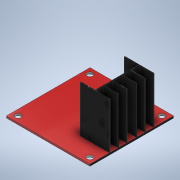
# Autodesk Inventor part: L298N
Saved by Autodesk Inventor 2022 (Build 260153000, 153)
## iProperties
Created: 2022-02-10
Part Number: L298N
Material: Generic
Document SubType Name: Modeling
Designer: matys
Density: 1 g/cm^3
Appearance: Default
Author: matys
Autodesk Inventor part; units mm, degrees
ref_plane "YZ Plane" through (0, 0, 0) normal (1, 0, 0) x (0, 1, 0)
ref_plane "XZ Plane" through (0, 0, 0) normal (0, 1, 0) x (-1, 0, 0)
ref_plane "XY Plane" through (0, 0, 0) normal (0, 0, 1) x (1, 0, 0)
sketch "Sketch1" plane through (0, 0, 0) normal (0, 1, 0) x (-1, 0, 0)
  line L0 (0, 0) -> (0, -43)
  line L1 (0, -43) -> (43, -43)
  line L2 (43, -43) -> (43, 0)
  line L3 (43, 0) -> (0, 0)
  dimension "d0" = 43
  dimension "d1" = 43
  constraints: 8 end point, 3 perpendicular, 1 vertical
  measures "d0" distance of L0.start L0.end
  measures "d1" distance of L0.end L1.end
extrude "Extrusion1" add sketch "Sketch1" along normal blind 1
sketch "Sketch2" plane through (0, 1, 0) normal (0, 1, 0) x (1, 0, 0)
  line L0 (-43, 0) -> (0, 0) projected
  line L1 (0, 0) -> (-3, 0)
  line L2 (-3, 0) -> (-3, 3)
  line L3 (-3, 3) -> (0, 3)
  circle A0 centre (-3, 3) radius 1.5
  line L4 (0, 43) -> (-43, 43) projected
  line L5 (0, 0) -> (-43, 43)
  line L6 (-43, 43) -> (-43, 0)
  line L7 (-43, 43) -> (-43, 0) projected
  line L8 (0, 0) -> (0, 43) projected
  line L9 (-43, 0) -> (0, 43)
  line L10 (0, 43) -> (-21.5, 21.5)
  circle A1 centre (-3, 40) radius 1.5
  circle A2 centre (-40, 40) radius 1.5
  circle A3 centre (-40, 3) radius 1.5
  dimension "d4" = 3
  dimension "d5" = 3
  dimension "d6" = 3
  dimension "d9" = 360
  constraints: 14 end point, 4 centre point, 4 perpendicular, 1 coincident, 1 midpoint, 1 point on line, 9 other
  measures "d4" distance of L0.end L1.end
  measures "d5" distance of L1.end L2.end
  measures "d6" diameter of A0
extrude "Extrusion2" cut sketch "Sketch2" against normal through all contours A3 L9 | L9 A3 | A0 L5 L2 | L2 L5 A0 | A2 L5 | L5 A2 | L5 L3 A0 | L5 A0 L3 | A1 L9 | L9 A1
sketch "Sketch3" plane through (0, 1, 0) normal (0, 1, 0) x (1, 0, 0)
  line L0 (-43, 0) -> (0, 0) projected
  line L1 (0, 0) -> (0, 10)
  line L2 (0, 0) -> (0, 43) projected
  line L3 (0, 10) -> (0, 43)
  line L4 (0, 43) -> (0, 33)
  line L5 (0, 33) -> (0, 10)
  line L6 (0, 10) -> (-15, 10)
  line L7 (-15, 10) -> (-15, 33)
  line L8 (-15, 33) -> (0, 33)
  line L9 (0, 10) -> (0, 14.4)
  line L10 (0, 14.4) -> (0, 18.8)
  line L11 (0, 33) -> (0, 28.6)
  line L12 (0, 28.6) -> (0, 24.2)
  line L13 (0, 24.2) -> (0, 18.8)
  line L14 (0, 14.4) -> (0, 15)
  line L15 (0, 33) -> (0, 32.6)
  line L16 (0, 32.6) -> (-15, 32.6)
  line L17 (0, 32.6) -> (0, 28.6)
  line L18 (0, 28.6) -> (-15, 28.6)
  line L19 (0, 28.6) -> (0, 28.2)
  line L20 (0, 28.2) -> (-15, 28.2)
  line L21 (0, 28.2) -> (0, 24.2)
  line L22 (0, 18.8) -> (0, 24.2)
  line L23 (0, 32.6) -> (0, 28.6)
  line L24 (0, 28.2) -> (0, 24.2)
  line L25 (0, 24.2) -> (-15, 24.2)
  line L26 (0, 24.2) -> (0, 23.8)
  line L27 (0, 23.8) -> (-15, 23.8)
  line L28 (0, 18.8) -> (0, 19.2)
  line L29 (0, 19.2) -> (-15, 19.2)
  line L30 (0, 18.8) -> (-15, 18.8)
  line L31 (0, 14.4) -> (-15, 14.4)
  line L32 (0, 10) -> (0, 10.4)
  line L33 (0, 10.4) -> (-15, 10.4)
  line L34 (0, 10.4) -> (0, 14.4)
  line L35 (0, 14.4) -> (0, 14.8)
  line L36 (0, 14.8) -> (-15, 14.8)
  line L37 (0, 10) -> (-7.5, 10)
  line L38 (-7.5, 10) -> (-7.5, 33)
  line L39 (-7.5, 10) -> (-7.7, 10)
  line L40 (-7.7, 10) -> (-7.3, 10)
  line L41 (-7.3, 10) -> (-7.3, 33)
  line L42 (-7.7, 10) -> (-7.7, 33)
  point P0 (-7.7, 10.4)
  point P1 (-7.3, 10.4)
  point P2 (-7.3, 14.4)
  point P3 (-7.3, 14.8)
  point P4 (-7.3, 18.8)
  point P5 (-7.3, 19.2)
  point P6 (-7.3, 23.8)
  point P7 (-7.3, 24.2)
  point P8 (-7.3, 28.2)
  point P9 (-7.3, 28.6)
  point P10 (-7.3, 32.6)
  point P11 (-7.7, 32.6)
  dimension "d13" = 10
  dimension "d14" = 10
  dimension "d15" = 23
  dimension "d16" = 15
  dimension "d17" = 4.4
  dimension "d18" = 4.4
  dimension "d19" = 4.4
  dimension "d20" = 4.4
  dimension "d22" = 0.4
  dimension "d23" = 0.4
  dimension "d24" = 0.4
  dimension "d25" = 0.4
  dimension "d26" = 0.4
  dimension "d27" = 0.4
  dimension "d28" = 0.2
  dimension "d29" = 0.4
  constraints: 80 end point, 17 point on line, 11 horizontal, 8 collinear, 5 perpendicular, 2 midpoint, 13 other
  measures "d13" distance of L0.end L1.end
  measures "d14" distance of L2.end L4.end
  measures "d15" distance of L4.end L1.end
  measures "d16" distance of L1.end L6.end
  measures "d17" distance of L1.end L9.end
  measures "d18" distance of L9.end L10.end
  measures "d19" distance of L4.end L11.end
  measures "d20" distance of L11.end L12.end
  measures "d22" distance of L4.end L15.end
  measures "d23" distance of L11.end L19.end
  measures "d24" distance of L12.end L26.end
  measures "d25" distance of L10.end L28.end
  measures "d26" distance of L1.end L32.end
  measures "d27" distance of L9.end L35.end
  measures "d28" distance of L37.end L39.end
  measures "d29" distance of L39.end L40.end
extrude "Extrusion3" add sketch "Sketch3" along normal blind 24 contours L6 L41 L33 L2 | L6 L38 L33 L41 | L31 L41 L36 L2 | L33 L38 L31 L41 | L6 L42 L33 L38 | L31 L38 L36 L41 | L33 L42 L31 L38 | L6 L7 L33 L42 | L36 L38 L30 L41 | L31 L42 L36 L38 | L30 L41 L29 L2 | L36 L42 L30 L38 | L30 L38 L29 L41 | L30 L42 L29 L38 | L29 L38 L27 L41 | L27 L41 L25 L2 | L29 L42 L27 L38 | L27 L38 L25 L41 | L27 L42 L25 L38 | L25 L38 L20 L41 | L20 L41 L18 L2 | L25 L42 L20 L38 | L20 L38 L18 L41 | L20 L42 L18 L38 | L18 L38 L16 L41 | L16 L41 L8 L2 | L18 L42 L16 L38 | L16 L38 L8 L41 | L16 L42 L8 L38 | L16 L7 L8 L42
body "Solid1"
